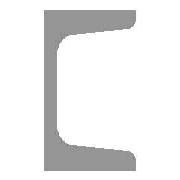
# Autodesk Inventor part: ISO 657/11 - CH 80 x 8 - 4800
Saved by Autodesk Inventor 2025 (Build 290162010, 162A)
## iProperties
Created: 2024-01-20
Part Number: ISO 657/11 - CH 80 x 8 - 4800
Material: Steel, Mild
Description: Hot rolled steel sloping flange channel sections
Document SubType Name: Modeling
Standard: ISO 657/11
Designer: admin
Standard Revision: First edition 1980-09-01
Standards Organization: ISO
Language: en-US
Size Designation: CH 80 x 8 - 4800
Categories: <MemberInstance><Categories><Category DisplayName="Structural Shapes" InternalName="089c4875-fa83-4c05-b084-43b9cc11f5ed" Mnemonic="GRDR"><CategoryParameter DisplayName="Mass per Length Unit" InternalName="0bb95a10-148f-4027-a459-38d7b056702a" Mnemonic="shpmass"/><CategoryParameter DisplayName="Section Area" InternalName="1ff91680-64b0-4202-b9a3-7fd3f94bba3b" Mnemonic="secarea"/><CategoryParameter DisplayName="Radius of Gyration (x)" InternalName="25778675-03e9-40c1-b6a8-4a9ed693320d" Mnemonic="gyrradx"/><CategoryParameter DisplayName="Torsional Rigidity Modulus" InternalName="26c1ec35-5026-4c63-ad0a-751cf684a536" Mnemonic="torrigmod"/><CategoryParameter DisplayName="Distance of the Center of Gravity X-X" InternalName="26c9bdb8-9c79-4b4f-a92e-8e197583c9c4" Mnemonic="grcendistX"/><CategoryParameter DisplayName="Legacy Member ID" InternalName="340afe4f-75d7-48d3-ab7d-943f3c3da468" Mnemonic="LegacyMemberID"/><CategoryParameter DisplayName="Base Length" InternalName="42e34263-8f20-4d0e-ad48-bf1385b87c24" Mnemonic="shplen"/><CategoryParameter DisplayName="Moment of Inertia (y)" InternalName="4b9f58ea-bced-460e-81ea-3d29ca5a49e3" Mnemonic="inermomy"/><CategoryParameter DisplayName="Moment of Inertia (x)" InternalName="4cd780bc-73d7-43ac-917a-579e5cbd684d" Mnemonic="inermomx"/><CategoryParameter DisplayName="Custom Base Point" InternalName="4f1d1b73-316d-484b-a3df-9cbabb16eb77" Mnemonic="shpBasePoint"/><CategoryParameter DisplayName="Shape Height" InternalName="50274e7d-5ac0-4796-92cb-c59e54983c67" Mnemonic="shpheig"/><CategoryParameter DisplayName="Section Module (y)" InternalName="59eaa5e9-d227-48dc-b6c1-6920f96e0f95" Mnemonic="secmody"/><CategoryParameter DisplayName="Section Designation" InternalName="5a64d034-428d-49c8-ba32-7619764de20f" Mnemonic="shpdes"/><CategoryParameter DisplayName="Section Module (x)" InternalName="72cfad18-cf51-4ed4-aaa7-c6b224f8419f" Mnemonic="secmodx"/><CategoryParameter DisplayName="Torsional Section Modulus" InternalName="7c55a8dc-8844-49f9-a867-cc677b30ec9a" Mnemonic="torsecmod"/><CategoryParameter DisplayName="Shape Width" InternalName="7c717d54-a18f-4666-b4d4-573cce22c62c" Mnemonic="shpwdth"/><CategoryParameter DisplayName="Second Shape Thickness" InternalName="9251a8e1-85fd-4e47-af99-afdb762317d9" Mnemonic="shpthick2"/><CategoryParameter DisplayName="FG Authored" InternalName="9c666724-f362-4ea7-ac62-f6a007de5c69" Mnemonic="shpFGAuto"/><CategoryParameter DisplayName="Distance of the Center of Gravity Y-Y" InternalName="bcc4fb17-7af4-436a-8f8c-d0aa3b0248c5" Mnemonic="grcendistY"/><CategoryParameter DisplayName="Radius of Gyration (y)" InternalName="bfa18ebe-1636-4dbe-8d42-b263e0b73184" Mnemonic="gyrrady"/><CategoryParameter DisplayName="Shape Thickness" InternalName="d109cf76-8eb4-42fc-9800-4409734adc67" Mnemonic="shpthick"/><CategoryParameter DisplayName="Coefficient of Shear Displacement" InternalName="de4c90c6-aaa8-468f-a335-6737b311b5d3" Mnemonic="shdispc"/><Category DisplayName="Channels" InternalName="afc9639c-904e-466f-b689-182c3a803db6" Mnemonic="USHP"><CategoryParameter DisplayName="Radius of Gyration (x)" InternalName="26fc5c1a-ceda-4f20-bae8-fdf59a032e92" Mnemonic="gyrradx"/><CategoryParameter DisplayName="Mass per Length Unit" InternalName="277ab211-d792-4c0c-bd86-88a051ce898e" Mnemonic="shpmass"/><CategoryParameter DisplayName="Moment of Inertia (x)" InternalName="629b89e9-88bd-407d-a4fb-8ed80285d9d3" Mnemonic="inermomx"/><CategoryParameter DisplayName="Shape Width" InternalName="72fdb865-5155-47d3-8635-1864da1bbc1e" Mnemonic="shpwdth"/><CategoryParameter DisplayName="Shape Thickness" InternalName="90483e77-719f-4576-adc3-8ddc4a7c3df5" Mnemonic="shpthick"/><CategoryParameter DisplayName="Radius of Gyration (y)" InternalName="b768ea18-1848-4f9a-b4e3-0277a85bba69" Mnemonic="gyrrady"/><CategoryParameter DisplayName="Section Module (x)" InternalName="bd40c05d-990f-41ce-9e17-ca66fb4811c6" Mnemonic="secmodx"/><CategoryParameter DisplayName="Moment of Inertia (y)" InternalName="c86e3d12-7670-41af-a3c5-3140b7cd40d5" Mnemonic="inermomy"/><CategoryParameter DisplayName="Second Shape Thickness" InternalName="db0066e2-a67f-4d9a-ab73-8cf1f2b64a3c" Mnemonic="shpthick2"/><CategoryParameter DisplayName="Section Area" InternalName="e17b7136-e82e-4ca9-a8af-d7502cd97fd0" Mnemonic="secarea"/><CategoryParameter DisplayName="Section Module (y)" InternalName="e5057e5f-6bca-4618-8c2b-f6e048154ab5" Mnemonic="secmody"/></Category></Category><Category DisplayName="DataType" InternalName="23b78d0f-2648-40c6-8793-ca6db495c9e8" Mnemonic="DATATYPE"><CategoryParameter DisplayName="DisplayName" InternalName="05415f3d-3907-474b-a020-eb9d644f4cf3" Mnemonic="DISPLAYNAME"/><CategoryParameter DisplayName="Standard" InternalName="0c0a119c-1e12-4c84-803f-101930972f5e" Mnemonic="STANDARD"/><CategoryParameter DisplayName="Description" InternalName="13903e3d-64b1-4950-80da-f627842ea37f" Mnemonic="DESCRIPTION"/><CategoryParameter DisplayName="Designation" InternalName="2675968c-4ce5-49e0-a4f5-552d29089031" Mnemonic="DESIGNATION"/><CategoryParameter DisplayName="Default Row" InternalName="2af9ec52-faaa-4026-b378-f9fa4afca842" Mnemonic="DEFAULTROW"/><CategoryParameter DisplayName="Folder Name" InternalName="3f06958e-8713-4116-9be7-ed6184ecc97b" Mnemonic="FOLDERNAME"/><CategoryParameter DisplayName="Revision Guid" InternalName="45a75005-10b1-4dfc-8d6d-dfe629f0b93c" Mnemonic="REVISIONGUID"/><CategoryParameter DisplayName="FileName" InternalName="8b46a4cc-9585-4fed-90c3-899f57e09a73" Mnemonic="FILENAME"/><CategoryParameter DisplayName="StdsOrg" InternalName="8f5914e1-4693-403f-8ab5-d37768198c9d" Mnemonic="STDSORG"/><CategoryParameter DisplayName="Family Version" InternalName="914462f6-6e19-4b14-ba84-155b9680b1d0" Mnemonic="FAMILYREVISION"/><CategoryParameter DisplayName="Standard Revision" InternalName="91d5a463-65c2-4fde-b823-3b7fea5e8e17" Mnemonic="STANDARDREVISION"/><CategoryParameter DisplayName="Member Revision" InternalName="a65d44b9-392f-4f4f-857b-e4b3d54996fe" Mnemonic="MEMBERREVISION"/><CategoryParameter DisplayName="ClipFormat" InternalName="bc51e27b-3422-4e78-93ef-cec197ddf230" Mnemonic="CLIPFORMAT"/><CategoryParameter DisplayName="Manufacturer" InternalName="cd6c7a72-a28a-4e50-99a9-2c7f4e13e5ad" Mnemonic="MANUFACTURER"/><CategoryParameter DisplayName="InternalName" InternalName="cf1d0246-76d9-4b4a-8305-fa0409afb5c1" Mnemonic="INTERNALNAME"/><CategoryParameter DisplayName="IsMetric" InternalName="e2385c5b-1ea4-4823-96a8-8de651266ec3" Mnemonic="ISMETRIC"/><Category DisplayName="Part" InternalName="c0e0b642-3bcb-4cc8-9e80-f96d35c4afa4" Mnemonic="PART"><CategoryParameter DisplayName="Part Number" InternalName="016b6077-bfbe-49bd-92c9-d8d59c39c941" Mnemonic="PARTNUMBER"/><CategoryParameter DisplayName="Stock Number" InternalName="4dba7c1c-e26c-444e-836c-b08b433409a8" Mnemonic="STOCKNUMBER"/><CategoryParameter DisplayName="Material Key" InternalName="5c9a8adb-dd2b-4535-b97f-0a94a95fe41f" Mnemonic="MATERIALKEY"/><CategoryParameter DisplayName="Material" InternalName="818a152a-d3c3-49ca-80ee-df7d91421b8e" Mnemonic="MATERIAL"/></Category></Category><Category DisplayName="Legacy Map DA" InternalName="924fff40-ddd0-4eff-ad42-30e3774ef79e" Mnemonic="LEGACYMAPDA"><CategoryParameter DisplayName="DACookie" InternalName="316934ee-8fe1-4c7a-9c36-f2d79e1add1a" Mnemonic="DACOOKIE"/></Category><Category DisplayName="LegacyMap" InternalName="cd87c42b-3e48-431e-b5c0-1cbeb14dfe77" Mnemonic="LEGACYMAP"><CategoryParameter DisplayName="unique DA member ID" InternalName="0918ad47-427f-4fed-ae26-24c81c58f590" Mnemonic="DACOOKIE"/><CategoryParameter DisplayName="Merge11 ID" InternalName="0ee8fb18-e2ed-4f39-96f6-1f4b5f50aa71" Mnemonic="MERGE11"/><CategoryParameter DisplayName="unique CC member ID" InternalName="5193edd4-b2b0-4ab4-9d54-de900eee34e0" Mnemonic="CCCOOKIE"/><CategoryParameter DisplayName="Split ID" InternalName="72b5c83c-be7f-45c4-ae51-9160ea6deb26" Mnemonic="SPLIT"/><CategoryParameter DisplayName="MemberID" InternalName="8e5e0294-fc51-4c8f-b3d7-003dc5ed94f6" Mnemonic="MEMBERID"/><CategoryParameter DisplayName="CatalogName" InternalName="d99d1e27-aa94-4de2-af4c-c348882a6f4f" Mnemonic="CATALOGNAME"/><CategoryParameter DisplayName="FamilyNumber" InternalName="e705e1f4-09cb-413e-91f9-551b4188271e" Mnemonic="FAMILYNUMBER"/></Category></Categories><FamilyTemplate Id="gp0101"><FamilyTemplateParameters><FamilyTemplateParameter ObjectType="kUserParameterObject" ValueType="xs:double" Id="1" ObjectReferenceKey="G_C"/><FamilyTemplateParameter ObjectType="kUserParameterObject" ValueType="xs:double" Id="3" ObjectReferenceKey="ex"/><FamilyTemplateParameter ObjectType="kUserParameterObject" ValueType="xs:double" Id="6" ObjectReferenceKey="B_L"/><FamilyTemplateParameter ObjectType="kUserParameterObject" ValueType="xs:double" Id="7" ObjectReferenceKey="G_IR"/><FamilyTemplateParameter ObjectType="kUserParameterObject" ValueType="xs:double" Id="9" ObjectReferenceKey="G_W"/><FamilyTemplateParameter ObjectType="kUserParameterObject" ValueType="xs:double" Id="10" ObjectReferenceKey="G_T"/><FamilyTemplateParameter ObjectType="kUserParameterObject" ValueType="xs:double" Id="11" ObjectReferenceKey="G_H"/><FamilyTemplateParameter ObjectType="kUserParameterObject" ValueType="xs:double" Id="13" ObjectReferenceKey="G_ER"/><FamilyTemplateParameter ObjectType="kUserParameterObject" ValueType="xs:double" Id="14" ObjectReferenceKey="G_T1"/><FamilyTemplateParameter ObjectType="kUserParameterObject" ValueType="xs:double" Id="15" ObjectReferenceKey="G_NG"/><FamilyTemplateParameter ObjectType="kPropertyObject" ValueType="xs:string" Id="100" ObjectReferenceKey="{32853F0F-3444-11d1-9E93-0060B03C1CA6}" SubObjectId="52"/><FamilyTemplateParameter ObjectType="kPropertyObject" ValueType="xs:string" Id="105" ObjectReferenceKey="{32853F0F-3444-11d1-9E93-0060B03C1CA6}" SubObjectId="5"/><FamilyTemplateParameter ObjectType="kPartComponentDefinitionObject" ValueType="xs:string" Id="110" SubObjectId="Material"/><FamilyTemplateParameter ObjectType="kPropertyObject" ValueType="xs:string" Id="112" ObjectReferenceKey="{32853F0F-3444-11d1-9E93-0060B03C1CA6}" SubObjectId="55"/></FamilyTemplateParameters></FamilyTemplate><CategoryParameterMap><ParamToTemplateMap><ParamToTemplate CategoryParameter="//CategoryParameter[@InternalName='05415f3d-3907-474b-a020-eb9d644f4cf3']" ConstantValue="ISO 657/11-1980(E)"/><ParamToTemplate CategoryParameter="//CategoryParameter[@InternalName='cf1d0246-76d9-4b4a-8305-fa0409afb5c1']" ConstantValue="a7a188dc-3195-43d7-8078-fd5c115750dc"/><ParamToTemplate CategoryParameter="//CategoryParameter[@InternalName='3f06958e-8713-4116-9be7-ed6184ecc97b']" ConstantValue="ISO 657 11 - 1980"/><ParamToTemplate CategoryParameter="//CategoryParameter[@InternalName='914462f6-6e19-4b14-ba84-155b9680b1d0']" ConstantValue="10"/><ParamToTemplate CategoryParameter="//CategoryParameter[@InternalName='bc51e27b-3422-4e78-93ef-cec197ddf230']" ConstantValue="CF_INVENTOR.STDPARTS"/><ParamToTemplate CategoryParameter="//CategoryParameter[@InternalName='e2385c5b-1ea4-4823-96a8-8de651266ec3']" ConstantValue="true"/><ParamToTemplate CategoryParameter="//CategoryParameter[@InternalName='13903e3d-64b1-4950-80da-f627842ea37f']" ConstantValue="Hot rolled steel sloping flange channel sections"/><ParamToTemplate CategoryParameter="//CategoryParameter[@InternalName='8f5914e1-4693-403f-8ab5-d37768198c9d']" ConstantValue="ISO"/><ParamToTemplate CategoryParameter="//CategoryParameter[@InternalName='0c0a119c-1e12-4c84-803f-101930972f5e']" ConstantValue="ISO 657/11"/><ParamToTemplate CategoryParameter="//CategoryParameter[@InternalName='cd6c7a72-a28a-4e50-99a9-2c7f4e13e5ad']" TemplateParameter="104"/><ParamToTemplate CategoryParameter="//CategoryParameter[@InternalName='91d5a463-65c2-4fde-b823-3b7fea5e8e17']" ConstantValue="First edition 1980-09-01"/><ParamToTemplate CategoryParameter="//CategoryParameter[@InternalName='45a75005-10b1-4dfc-8d6d-dfe629f0b93c']" ConstantValue="3f881134-343b-4304-9f96-47269fa3f422"/><ParamToTemplate CategoryParameter="//CategoryParameter[@InternalName='2af9ec52-faaa-4026-b378-f9fa4afca842']" ConstantValue="1"/><ParamToTemplate CategoryParameter="//CategoryParameter[@InternalName='9c666724-f362-4ea7-ac62-f6a007de5c69']" ConstantValue="1"/><ParamToTemplate CategoryParameter="//CategoryParameter[@InternalName='d99d1e27-aa94-4de2-af4c-c348882a6f4f']" ConstantValue="ISO"/><ParamToTemplate CategoryParameter="//CategoryParameter[@InternalName='e705e1f4-09cb-413e-91f9-551b4188271e']" ConstantValue="149"/><ParamToTemplate CategoryParameter="//CategoryParameter[@InternalName='8b46a4cc-9585-4fed-90c3-899f57e09a73']" ConstantValue="ISO 657/11 - CH 80 x 8 - 4800"/><ParamToTemplate CategoryParameter="//CategoryParameter[@InternalName='a65d44b9-392f-4f4f-857b-e4b3d54996fe']" ConstantValue="8B34943D-369B-4D90-A4D4-E9A0E3CC7B5D"/><ParamToTemplate CategoryParameter="//CategoryParameter[@InternalName='629b89e9-88bd-407d-a4fb-8ed80285d9d3']" ConstantValue="102"/><ParamToTemplate CategoryParameter="//CategoryParameter[@InternalName='c86e3d12-7670-41af-a3c5-3140b7cd40d5']" ConstantValue="18"/><ParamToTemplate CategoryParameter="//CategoryParameter[@InternalName='bd40c05d-990f-41ce-9e17-ca66fb4811c6']" ConstantValue="25,6"/><ParamToTemplate CategoryParameter="//CategoryParameter[@InternalName='e5057e5f-6bca-4618-8c2b-f6e048154ab5']" ConstantValue="5,85"/><ParamToTemplate CategoryParameter="//CategoryParameter[@InternalName='7c55a8dc-8844-49f9-a867-cc677b30ec9a']" ConstantValue="3370,4704"/><ParamToTemplate CategoryParameter="//CategoryParameter[@InternalName='26c1ec35-5026-4c63-ad0a-751cf684a536']" ConstantValue="18537,587"/><ParamToTemplate CategoryParameter="//CategoryParameter[@InternalName='e17b7136-e82e-4ca9-a8af-d7502cd97fd0']" ConstantValue="10,5"/><ParamToTemplate CategoryParameter="//CategoryParameter[@InternalName='de4c90c6-aaa8-468f-a335-6737b311b5d3']" ConstantValue="2"/><ParamToTemplate CategoryParameter="//CategoryParameter[@InternalName='26fc5c1a-ceda-4f20-bae8-fdf59a032e92']" ConstantValue="3,12"/><ParamToTemplate CategoryParameter="//CategoryParameter[@InternalName='b768ea18-1848-4f9a-b4e3-0277a85bba69']" ConstantValue="1,3"/><ParamToTemplate CategoryParameter="//CategoryParameter[@InternalName='5a64d034-428d-49c8-ba32-7619764de20f']" ConstantValue="CH 80 x 8"/><ParamToTemplate CategoryParameter="//CategoryParameter[@InternalName='8e5e0294-fc51-4c8f-b3d7-003dc5ed94f6']" ConstantValue="1"/><ParamToTemplate CategoryParameter="//CategoryParameter[@InternalName='316934ee-8fe1-4c7a-9c36-f2d79e1add1a']" ConstantValue="*ISO~N425571~CH  80 x  8*"/><ParamToTemplate CategoryParameter="//CategoryParameter[@InternalName='42e34263-8f20-4d0e-ad48-bf1385b87c24']" TemplateParameter="6"/><ParamToTemplate CategoryParameter="//CategoryParameter[@InternalName='2675968c-4ce5-49e0-a4f5-552d29089031']" TemplateParameter="100"/><ParamToTemplate CategoryParameter="//CategoryParameter[@InternalName='50274e7d-5ac0-4796-92cb-c59e54983c67']" TemplateParameter="11"/><ParamToTemplate CategoryParameter="//CategoryParameter[@InternalName='818a152a-d3c3-49ca-80ee-df7d91421b8e']" TemplateParameter="110"/><ParamToTemplate CategoryParameter="//CategoryParameter[@InternalName='016b6077-bfbe-49bd-92c9-d8d59c39c941']" TemplateParameter="105"/><ParamToTemplate CategoryParameter="//CategoryParameter[@InternalName='4dba7c1c-e26c-444e-836c-b08b433409a8']" TemplateParameter="112"/><ParamToTemplate CategoryParameter="//CategoryParameter[@InternalName='26c9bdb8-9c79-4b4f-a92e-8e197583c9c4']" TemplateParameter="3"/></ParamToTemplateMap></CategoryParameterMap></MemberInstance>
Stock Number: CH 80 x 8
Density: 7.85 g/cm^3
Appearance: Semi-Polished
G_L: 4800,000 mm
IsCustomPart: 1
Author: admin
Autodesk Inventor part; units mm, degrees
ref_plane "YZ Plane" through (0, 0, 0) normal (1, 0, 0) x (0, 1, 0)
ref_plane "Start plane" through (0, 0, 0) normal (0, 0, 1) x (1, 0, 0)
ref_plane "End plane" through (0, 0, 4800) normal (0, 0, 1) x (1, 0, 0)
sketch "Sketch" plane through (0, 0, 0) normal (0, 0, 1) x (1, 0, 0)
  line L0 (-1.43, 0) -> (-1.43, 40)
  line L1 (-1.43, 40) -> (43.57, 40)
  line L2 (43.57, 40) -> (43.57, 38.1774)
  line L3 (39.9881, 34.1993) -> (11.2338, 31.1771)
  line L4 (4.07, 23.221) -> (4.07, 0)
  line L5 (4.07, 0) -> (-1.43, 0) construction
  line L6 (23.82, 40) -> (23.82, 32.5) construction
  line L7 (43.57, 34.5758) -> (43.57, 32.5) construction
  line L8 (43.57, 32.5) -> (23.82, 32.5) construction
  line L9 (0, 15) -> (0, -27) construction
  line L10 (-5.539, 0) -> (16.0067, 0) construction
  line L11 (-1.43, 0) -> (-1.43, -40)
  line L12 (-1.43, -40) -> (43.57, -40)
  line L13 (43.57, -40) -> (43.57, -38.1774)
  line L14 (39.9881, -34.1993) -> (11.2338, -31.1771)
  line L15 (4.07, -23.221) -> (4.07, 0)
  arc A0 (11.2338, 31.1771) -> (4.07, 23.221) centre (12.07, 23.221) ccw
  arc A1 (4.07, -23.221) -> (11.2338, -31.1771) centre (12.07, -23.221) ccw
  arc A2 (39.9881, 34.1993) -> (43.57, 38.1774) centre (39.57, 38.1774) ccw
  arc A3 (43.57, -38.1774) -> (39.9881, -34.1993) centre (39.57, -38.1774) ccw
  line L16 (0, 23.4) -> (0, -35.4) construction
  line L17 (-9.8481, 0) -> (20.3158, 0) construction
  point P0 (4.07, 30.4242)
  point P1 (43.57, -34.5758)
  point P2 (4.07, -30.4242)
  point P3 (23.82, -40)
  point P4 (23.82, -32.5)
  dimension "d0" = 5.5
  dimension "d1" = 40
  dimension "d2" = 45
  dimension "d3" = 7.5
  dimension "d4" = 19.75
  dimension "d5" = 2.0758
  dimension "d23" = 8
  dimension "d24" = 4
  dimension "d25" = 1.43
  constraints: 32 end point, 12 point on line, 8 point on circle, 8 tangent, 6 symmetric about line, 4 centre point, 4 parallel, 3 collinear, 3 perpendicular, 2 equal radius, 5 other
  measures "d0" distance between parallel lines of L0 L4
  measures "d1" distance between parallel lines of L5 L1
  measures "d2" distance between parallel lines of L2 L0
  measures "d3" distance of L1.end L7.end
  measures "d4" distance of L6.start L1.end
  measures "d5" distance of L7.start L7.end
  measures "d23" radius of A0
  measures "d24" radius of A2
  measures "d25" distance between parallel lines of L9 L11
extrude "Body" add sketch "Sketch" along normal up to surface (4800 mm away) from surface at 0
sketch "Sketch3" plane through (0, 0, 0) normal (0, 0, 1) x (1, 0, 0)
  line L0 (0, 0) -> (10, 0)
ref_plane "Work Plane3" through (0, 0, 0) normal (0, -1, 0) x (1, 0, 0)
sketch "Sketch4" plane through (0, 0, 0) normal (0, -1, 0) x (1, 0, 0)
  line L0 (-2, 0) -> (12, 0) projected
  line L1 (-2, 4800) -> (12, 4800) projected
  dimension "d29" = 4800
  measures "d29" distance between parallel lines of L0 L1
equation "\"d0\" = G_T"
equation "\"d1\" = 0.5 * G_H"
equation "\"d2\" = G_W"
equation "\"d3\" = G_T1"
equation "\"d4\" = G_C"
equation "\"d23\" = G_IR"
equation "\"d24\" = G_ER"
equation "\"d25\" = ex"
equation "\"d6\" = G_L"
equation "\"G_W\" = 45"
equation "\"G_T\" = 5.5"
equation "\"G_T1\" = 7.5"
equation "\"G_NG\" = 0.105104"
equation "\"G_ER\" = 4"
equation "\"G_IR\" = 8"
equation "\"G_C\" = 19.75"
equation "\"G_L\" = d29"
equation "\"ex\" = 1.43"
equation "\"G_OFFSET_START\" = 0"
equation "\"G_OFFSET_END\" = 0"
equation "\"G_H\" = 80"
body "Solid1"
